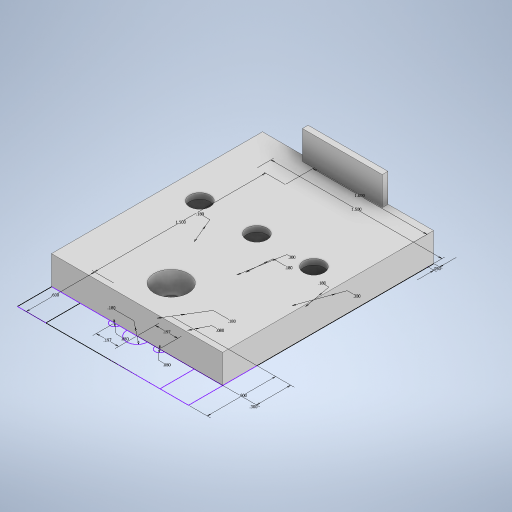
# Autodesk Inventor part: BeamsplitterMounttoPolarisPinAdapterV3
Saved by Autodesk Inventor 2024.2 (Build 282272000, 272)
## iProperties
Created: 2024-02-07
Part Number: BeamsplitterMounttoPolarisPinAdapterV3
Material: Generic
Document SubType Name: Modeling
Designer: monolithic
Density: 1 g/cm^3
Appearance: Default
Author: monolithic
Autodesk Inventor part; units mm, degrees
ref_plane "YZ Plane" through (0, 0, 0) normal (1, 0, 0) x (0, 1, 0)
ref_plane "XZ Plane" through (0, 0, 0) normal (0, 1, 0) x (-1, 0, 0)
ref_plane "XY Plane" through (0, 0, 0) normal (0, 0, 1) x (1, 0, 0)
sketch "Sketch1" plane through (0, 0, 0) normal (0, 1, 0) x (-1, 0, 0)
  line L0 (-12.7, 19.05) -> (12.7, 19.05)
  line L1 (12.7, 19.05) -> (12.7, -19.05)
  line L2 (12.7, -19.05) -> (-12.7, -19.05)
  line L3 (-12.7, -19.05) -> (-12.7, 19.05)
  line L4 (-12.7, 19.05) -> (12.7, -19.05) construction
  line L5 (12.7, 19.05) -> (-12.7, -19.05) construction
  circle A0 centre (0, 0) radius 2.286
  line L6 (12.7, 19.05) -> (-12.7, 19.05)
  line L7 (-12.7, 19.05) -> (-12.7, 34.29)
  line L8 (-12.7, 34.29) -> (12.7, 34.29)
  line L9 (12.7, 34.29) -> (12.7, 19.05)
  line L10 (-19.05, 19.05) -> (19.05, 19.05)
  line L11 (19.05, 19.05) -> (19.05, -19.05)
  line L12 (19.05, -19.05) -> (-19.05, -19.05)
  line L13 (-19.05, -19.05) -> (-19.05, 19.05)
  line L14 (-19.05, 19.05) -> (19.05, -19.05) construction
  line L15 (19.05, 19.05) -> (-19.05, -19.05) construction
  circle A1 centre (12.7, 0) radius 2.286
  circle A2 centre (-12.7, 0) radius 2.286
  line L16 (19.05, 19.05) -> (-19.05, 19.05)
  line L17 (-19.05, 19.05) -> (-19.05, 34.29)
  line L18 (-19.05, 34.29) -> (19.05, 34.29)
  line L19 (19.05, 34.29) -> (19.05, 19.05)
  circle A3 centre (0, 26.67) radius 2.286
  line L20 (-19.05, -19.05) -> (19.05, -19.05)
  line L21 (19.05, -19.05) -> (19.05, -20.32)
  line L22 (19.05, -20.32) -> (-19.05, -20.32)
  line L23 (-19.05, -20.32) -> (-19.05, -19.05)
  circle A4 centre (0, 0) radius 3.81
  circle A5 centre (-12.7, 0) radius 3.81
  circle A6 centre (12.7, 0) radius 3.81
  line L24 (0, 26.67) -> (-5.0038, 26.67)
  line L25 (-5.0038, 26.67) -> (0, 26.67)
  line L26 (0, 26.67) -> (5.0038, 26.67)
  circle A7 centre (5.0038, 26.67) radius 1.016
  circle A8 centre (-5.0038, 26.67) radius 1.016
  circle A9 centre (0, 19.05) radius 2.286
  circle A10 centre (-5.0038, 19.05) radius 1.016
  circle A11 centre (5.0038, 19.05) radius 1.016
  line L27 (-19.05, 26.67) -> (19.05, 26.67)
  point P0 (12.7, 34.29)
  dimension "d0" = 38.1
  dimension "d1" = 25.4
  dimension "d2" = 4.572
  dimension "d3" = 15.24
  dimension "d4" = 38.1
  dimension "d5" = 4.572
  dimension "d6" = 4.572
  dimension "d7" = 4.572
  dimension "d10" = 1.27
  dimension "d13" = 15.24
  dimension "d14" = 7.62
  dimension "d15" = 7.62
  dimension "d16" = 7.62
  dimension "d22" = 5.0038
  dimension "d23" = 5.0038
  dimension "d24" = 2.032
  dimension "d25" = 2.032
  dimension "d28" = 4.572
  dimension "d29" = 2.032
  constraints: 56 end point, 12 centre point, 11 equal length, 9 midpoint, 7 coincident, 6 horizontal, 5 perpendicular, 3 point on line
  measures "d0" distance of L0.end L1.end
  measures "d1" distance of L1.end L2.end
  measures "d2" diameter of A0
  measures "d3" distance of L8.end L0.end
  measures "d4" distance of L11.end L12.end
  measures "d5" diameter of A1
  measures "d6" diameter of A2
  measures "d7" diameter of A3
  measures "d10" distance of L22.end L12.end
  measures "d13" distance of L16.end L17.end
  measures "d14" distance of point (0, 19.05) L24.start
  measures "d15" diameter of A4
  measures "d16" diameter of A5
  measures "d22" distance of L24.start L24.end
  measures "d23" distance of L24.start L26.end
  measures "d24" diameter of A7
  measures "d25" diameter of A8
  measures "d28" diameter of A9
  measures "d29" diameter of A10
extrude "Extrusion1" add sketch "Sketch1" along normal blind 6.35 contours A11 L0 A9 A10 L7 L27 A8 L24 A3 L26 A7 L9 | A11 L0 | L0 A11 | L0 L1 A6 L2 L3 A5 A10 A9 A11 | L10 L11 L12 L1 A6 | L9 L27 L19 L10 | A6 L1 A1 | L1 A1 A6 | A7 L26 L27 | A10 L0 | L0 A10 | L12 L13 L10 L3 A5 | L7 L10 L17 L27 | A3 L24 L26 | A5 L3 A2 | L3 A2 A5 | L27 L24 A8 | A4 picked at (4.3363, 26.589) picked at (-1.5019, 26.4876) picked at (-5.6713, 26.589)
extrude "Extrusion2" add sketch "Sketch1" along normal blind 12.7 contours L21 L22 L23 L12 L2
extrude "Extrusion3" cut sketch "Sketch1" along normal blind 5.08 contours A6 L1 A1 | L1 A1 A6 | A5 L3 A2 | L3 A2 A5 | A4
sketch "Sketch2" plane through (0, 6.35, 0) normal (0, 1, 0) x (1, 0, 0)
  circle A0 centre (0, -26.67) radius 2.286 projected
  circle A1 centre (0, -26.67) radius 3.81
  circle A2 centre (0, -19.0503) radius 3.81
  point P0 (0, 0)
  point P1 (0.035, -22.8602)
  point P2 (-0.035, -22.8602)
  dimension "d19" = 7.62
  constraints: 2 centre point, 1 coincident
  measures "d19" diameter of A1
extrude "Extrusion4" cut sketch "Sketch2" against normal blind 5.08 contours A2
sketch "Sketch3" plane through (0, 0, 0) normal (0, -1, 0) x (1, 0, 0)
  point P0 (0, 0)
extrude "Extrusion5" cut sketch "Sketch1" along normal blind 4.445 contours A11 L0 | L0 A11 | A10 L0 | L0 A10
sketch "Sketch4" plane through (19.05, 0, -20.32) normal (0, 0, -1) x (-1, 0, 0)
  point P0 (19.05, 0)
sketch "Sketch5" plane through (-19.05, 6.35, -19.05) normal (0, 0, 1) x (1, 0, 0)
  line L0 (38.1, 6.35) -> (0, 6.35) projected
  line L1 (0, 6.35) -> (10.16, 6.35)
  line L2 (10.16, 6.35) -> (10.16, 0)
  line L3 (10.16, 0) -> (0, 0)
  line L4 (0, 0) -> (0, 6.35)
  line L5 (0, 0) -> (38.1, 0) projected
  line L6 (38.1, 6.35) -> (27.94, 6.35)
  line L7 (27.94, 6.35) -> (27.94, 0)
  line L8 (27.94, 0) -> (38.1, 0)
  line L9 (38.1, 0) -> (38.1, 6.35)
  point P0 (19.05, -6.35)
  dimension "d30" = 10.16
  dimension "d31" = 10.16
  dimension "d32" = 6.35
  constraints: 16 end point, 4 parallel, 2 horizontal, 2 perpendicular, 2 point on line
  measures "d30" distance of L2.end L3.end
  measures "d31" distance of L8.end L7.end
  measures "d32" distance of L3.end L0.end
extrude "Extrusion6" cut sketch "Sketch5" against normal blind 25.4 contours L9 L5 L7 L0 | L2 L3 L4 L0
body "Solid1"
